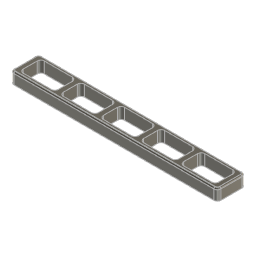
gridfinity_alex_drawerspacer (Autodesk Fusion 360 design; units mm, degrees)
Autodesk Fusion 360 part; units mm, degrees
sketch "Sketch1" plane through (0, 0, 0) normal (0, 0, 1) x (1, 0, 0)
  line L0 (0, 0) -> (147, 0)
  line L1 (147, 0) -> (147, 20)
  line L2 (147, 20) -> (0, 20)
  line L3 (0, 20) -> (0, 0)
  line L4 (6.5, 17.5) -> (26.5, 17.5)
  line L5 (29, 15) -> (29, 5)
  line L6 (26.5, 2.5) -> (6.5, 2.5)
  line L7 (4, 5) -> (4, 15)
  line L8 (147, 10) -> (0, 10) construction
  line L9 (4, 10) -> (29, 10) construction
  line L10 (35, 17.5) -> (55, 17.5)
  line L11 (32.5, 5) -> (32.5, 15)
  line L12 (57.5, 15) -> (57.5, 5)
  line L13 (55, 2.5) -> (35, 2.5)
  line L14 (63.5, 17.5) -> (83.5, 17.5)
  line L15 (61, 5) -> (61, 15)
  line L16 (86, 15) -> (86, 5)
  line L17 (83.5, 2.5) -> (63.5, 2.5)
  line L18 (92, 17.5) -> (112, 17.5)
  line L19 (89.5, 5) -> (89.5, 15)
  line L20 (114.5, 15) -> (114.5, 5)
  line L21 (112, 2.5) -> (92, 2.5)
  line L22 (120.5, 17.5) -> (140.5, 17.5)
  line L23 (118, 5) -> (118, 15)
  line L24 (143, 15) -> (143, 5)
  line L25 (140.5, 2.5) -> (120.5, 2.5)
  arc A0 (6.5, 17.5) -> (4, 15) centre (6.5, 15) ccw
  arc A1 (4, 5) -> (6.5, 2.5) centre (6.5, 5) ccw
  arc A2 (26.5, 2.5) -> (29, 5) centre (26.5, 5) ccw
  arc A3 (29, 15) -> (26.5, 17.5) centre (26.5, 15) ccw
  arc A4 (35, 17.5) -> (32.5, 15) centre (35, 15) ccw
  arc A5 (32.5, 5) -> (35, 2.5) centre (35, 5) ccw
  arc A6 (55, 2.5) -> (57.5, 5) centre (55, 5) ccw
  arc A7 (57.5, 15) -> (55, 17.5) centre (55, 15) ccw
  arc A8 (63.5, 17.5) -> (61, 15) centre (63.5, 15) ccw
  arc A9 (61, 5) -> (63.5, 2.5) centre (63.5, 5) ccw
  arc A10 (83.5, 2.5) -> (86, 5) centre (83.5, 5) ccw
  arc A11 (86, 15) -> (83.5, 17.5) centre (83.5, 15) ccw
  arc A12 (92, 17.5) -> (89.5, 15) centre (92, 15) ccw
  arc A13 (89.5, 5) -> (92, 2.5) centre (92, 5) ccw
  arc A14 (112, 2.5) -> (114.5, 5) centre (112, 5) ccw
  arc A15 (114.5, 15) -> (112, 17.5) centre (112, 15) ccw
  arc A16 (120.5, 17.5) -> (118, 15) centre (120.5, 15) ccw
  arc A17 (118, 5) -> (120.5, 2.5) centre (120.5, 5) ccw
  arc A18 (140.5, 2.5) -> (143, 5) centre (140.5, 5) ccw
  arc A19 (143, 15) -> (140.5, 17.5) centre (140.5, 15) ccw
  point P0 (4, 17.5)
  point P1 (29, 17.5)
  point P2 (4, 2.5)
  dimension "d1" = 147
  dimension "d2" = 20
  dimension "d5" = 25
  dimension "d6" = 15
  dimension "d11" = 4
  dimension "d12" = 2.5
  dimension "d13" = 2.5
  constraint horizontal L0
  constraint vertical L1
  constraint horizontal L2
  constraint vertical L3
  constraint coincident L0.start L3.end
  constraint horizontal L4
  constraint vertical L5
  constraint horizontal L6
  constraint vertical L7
  constraint midpoint L1 L8.start
  constraint midpoint L3 L8.end
  constraint collinear L8 L9
  constraint coincident L7 L9.start
  constraint coincident P0 L4
  constraint coincident P0 L7
  constraint tangent L4 A0
  constraint tangent L7 A0
  constraint coincident P2 L7
  constraint coincident P2 L6
  constraint tangent L7 A1
  constraint tangent L6 A1
  constraint equal A0 A1
  constraint coincident L5 L9.end
  constraint tangent L6 A2
  constraint tangent L5 A2
  constraint equal A0 A2
  constraint coincident P1 L5
  constraint coincident P1 L4
  constraint tangent L5 A3
  constraint tangent L4 A3
  constraint equal A0 A3
  constraint tangent L10 A4
  constraint tangent L11 A4
  constraint tangent L11 A5
  constraint tangent L13 A5
  constraint equal A4 A5
  constraint tangent L12 A6
  constraint tangent L13 A6
  constraint equal A4 A6
  constraint tangent L12 A7
  constraint tangent L10 A7
  constraint equal A4 A7
  constraint tangent L14 A8
  constraint tangent L15 A8
  constraint equal A4 A8
  constraint tangent L15 A9
  constraint tangent L17 A9
  constraint equal A4 A9
  constraint tangent L17 A10
  constraint tangent L16 A10
  constraint equal A4 A10
  constraint tangent L16 A11
  constraint tangent L14 A11
  constraint equal A4 A11
  constraint tangent L18 A12
  constraint tangent L19 A12
  constraint equal A4 A12
  constraint tangent L19 A13
  constraint tangent L21 A13
  constraint equal A4 A13
  constraint tangent L21 A14
  constraint tangent L20 A14
  constraint equal A4 A14
  constraint tangent L20 A15
  constraint tangent L18 A15
  constraint equal A4 A15
  constraint tangent L23 A16
  constraint tangent L22 A16
  constraint equal A4 A16
  constraint tangent L23 A17
  constraint tangent L25 A17
  constraint equal A4 A17
  constraint tangent L25 A18
  constraint tangent L24 A18
  constraint equal A4 A18
  constraint tangent L24 A19
  constraint tangent L22 A19
  constraint equal A4 A19
  measures "d1" distance of L1.end L2.end
  measures "d2" distance of L0.start L2.end
  measures "d5" distance of P0 P1
  measures "d6" distance of P0 P2
  measures "d11" distance of L3 L7
  measures "d12" radius of A0
  measures "d13" radius of A4
extrude "Extrude1" add sketch "Sketch1" along normal blind 8
fillet "Fillet1" radius 2.5 4 edges at (0, 0, 4) (0, 20, 4) (147, 0, 4) (147, 20, 4)
fillet "Fillet2" radius 1 8 edges at (146.2678, 0.7322, 8) (147, 10, 8) (146.2678, 19.2678, 8) (73.5, 20, 8) (0.7322, 19.2678, 8) (0, 10, 8) (0.7322, 0.7322, 8) (73.5, 0, 8)
equation "d1 = ( ( 42 * 7 ) / 2 ) * 1 mm"
named bodies: "gridfinity_spacer_ikea_alex"
